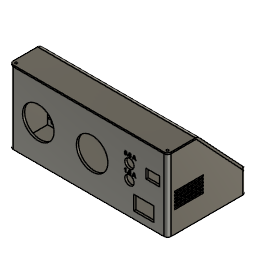
Darkroom timer box (Autodesk Fusion 360 design; units mm, degrees)
Autodesk Fusion 360 part; units mm, degrees
sketch "Sketch1" plane through (0, 0, 0) normal (0, 0, 1) x (1, 0, 0)
  line L0 (50, 125) -> (210, 125) construction
  line L1 (210, 125) -> (210, 25) construction
  line L2 (210, 25) -> (50, 25) construction
  line L3 (50, 25) -> (50, 125) construction
  line L4 (49, 225) -> (121, 225) construction
  line L5 (121, 225) -> (121, 224) construction
  line L6 (121, 224) -> (49, 224) construction
  line L7 (49, 224) -> (49, 225) construction
  line L8 (59, 224) -> (111, 224) construction
  line L9 (111, 224) -> (111, 192) construction
  line L10 (111, 192) -> (59, 192) construction
  line L11 (59, 192) -> (59, 224) construction
  line L12 (42, 225) -> (128, 225) construction
  line L13 (128, 225) -> (128, 237) construction
  line L14 (128, 237) -> (42, 237) construction
  line L15 (42, 237) -> (42, 225) construction
  line L16 (85, 240) -> (85, 190)
  line L17 (40, 130) -> (260, 130)
  line L18 (260, 130) -> (260, 20)
  line L19 (260, 20) -> (40, 20)
  line L20 (40, 20) -> (40, 130)
  line L21 (43, 127) -> (257, 127)
  line L22 (257, 127) -> (257, 23)
  line L23 (257, 23) -> (43, 23)
  line L24 (43, 23) -> (43, 127)
  line L25 (43, 115) -> (43, 120)
  line L26 (135, 120) -> (125, 120)
  line L27 (125, 120) -> (125, 127)
  line L28 (125, 127) -> (135, 127)
  line L29 (135, 127) -> (135, 120)
  line L30 (125, 30) -> (135, 30)
  line L31 (135, 30) -> (135, 23)
  line L32 (135, 23) -> (125, 23)
  line L33 (125, 23) -> (125, 30)
  line L34 (43, 35) -> (43, 30)
  line L35 (135, 126) -> (125, 126)
  line L36 (135, 24) -> (125, 24)
  circle A0 centre (44.5, 125.5) radius 1.5
  circle A1 centre (44.5, 125.5) radius 4
  circle A2 centre (255.5, 125.5) radius 1.5
  circle A3 centre (255.5, 125.5) radius 4
  line L37 (361, 251.0202) -> (361, 2.9798)
  circle A4 centre (44.5, 24.5) radius 1.5
  circle A5 centre (44.5, 24.5) radius 4
  circle A6 centre (255.5, 24.5) radius 1.5
  circle A7 centre (255.5, 24.5) radius 4
  line L38 (361, 150.0202) -> (361, -98.0202)
  line L39 (205, 70) -> (215, 70)
  line L40 (215, 70) -> (215, 80)
  line L41 (215, 80) -> (205, 80)
  line L42 (205, 80) -> (205, 70)
  line L43 (55, 70) -> (43, 70)
  line L44 (43, 70) -> (43, 80)
  line L45 (43, 80) -> (55, 80)
  line L46 (55, 80) -> (55, 70)
  line L47 (48, 70) -> (48, 80)
  line L48 (211, 70) -> (211, 80)
  point P0 (150, 75)
  dimension "d1" = 160
  dimension "d2" = 100
  dimension "d10" = 3
  dimension "d11" = 220
  dimension "d12" = 110
  constraint horizontal L0
  constraint vertical L1
  constraint horizontal L2
  constraint vertical L3
  constraint horizontal L4
  constraint vertical L5
  constraint horizontal L6
  constraint vertical L7
  constraint horizontal L8
  constraint vertical L9
  constraint horizontal L10
  constraint vertical L11
  constraint coincident L6 L8.start
  constraint horizontal L12
  constraint vertical L13
  constraint horizontal L14
  constraint vertical L15
  constraint perpendicular L10 L16
  constraint horizontal L17
  constraint vertical L18
  constraint horizontal L19
  constraint vertical L20
  constraint vertical L25
  constraint coincident L24 L25.end
  constraint horizontal L26
  constraint vertical L27
  constraint horizontal L28
  constraint vertical L29
  constraint coincident L21 L27.end
  constraint horizontal L30
  constraint vertical L31
  constraint horizontal L32
  constraint vertical L33
  constraint coincident L23 L31.end
  constraint vertical L34
  constraint coincident L24 L34.end
  constraint coincident L29 L35.start
  constraint coincident L27 L35.end
  constraint perpendicular L27 L35
  constraint coincident L31 L36.start
  constraint coincident L33 L36.end
  constraint perpendicular L33 L36
  constraint horizontal L39
  constraint vertical L40
  constraint horizontal L41
  constraint vertical L42
  constraint horizontal L43
  constraint vertical L44
  constraint horizontal L45
  constraint vertical L46
  constraint coincident L24 L44.end
  constraint coincident L45 L47.end
  constraint perpendicular L45 L47
  constraint coincident L39 L48.start
  constraint coincident L41 L48.end
  constraint perpendicular L41 L48
  measures "d1" distance of L0.start L0.end
  measures "d2" distance of L0.start L2.end
  measures "d11" distance of L17.start L17.end
  measures "d12" distance of L17.start L19.end
extrude "Extrude1" add sketch "Sketch1" along normal blind 4 contours L17 L18 L19 L20 | L21 L22 L23 L24 L25 L26 L27 L29 L30 L31 L33 L34 A1 A3 A5 A7 L43 L45 L46 | L21 L27 L28 L29 L35 | L21 L24 A0 A1 | L21 L24 A1 | L26 L27 L29 L35 | L21 L22 A3 | L21 L22 A2 A3 | L21 L24 A0 | A0 | L21 L22 A2 | A2 | L22 L23 A7 | L22 L23 A6 A7 | A6 | L22 L23 A6 | L24 L43 L44 L45 L47 | L23 L31 L32 L33 L36 | L43 L45 L46 L47 | L30 L31 L33 L36 | L23 L24 A5 | L23 L24 A4 A5 | L23 L24 A4 | A4 | L39 L41 L42 L48 | L39 L40 L41 L48 makes body 1
extrude "Extrude2" add sketch "Sketch1" along normal blind 100 contours L17 L18 L19 L20 | L21 L24 A0 A1 | L21 L24 A1 | L21 L22 A3 | L21 L22 A2 A3 | L21 L24 A0 | L21 L22 A2 | L22 L23 A7 | L22 L23 A6 A7 | L22 L23 A6 | L23 L24 A5 | L23 L24 A4 A5 | L23 L24 A4 bodies 1
extrude "Extrude3" add sketch "Sketch1" along normal blind 8 from surface at 4 contours L21 L27 L28 L29 L35 | L24 L43 L44 L45 L47 | L23 L31 L32 L33 L36 | L39 L40 L41 L48 bodies 1
extrude "Extrude5" add sketch "Sketch1" along normal blind 4 from surface at 4 contours L26 L27 L29 L35 | L43 L45 L46 L47 | L30 L31 L33 L36 | L39 L41 L42 L48 bodies 1
sketch "Sketch2" plane through (0, 20, 0) normal (0, -1, 0) x (1, 0, 0)
  line L0 (40, 0) -> (260, 0)
  line L1 (260, 0) -> (260, 100)
  line L2 (40, 100) -> (40, 0)
  circle A0 centre (80, 50) radius 22
  line L3 (45, 15) -> (45, 85)
  line L4 (45, 85) -> (115, 85)
  line L5 (115, 15) -> (45, 15)
  line L6 (115, 85) -> (115, 15)
  circle A1 centre (155, 50) radius 22
  line L7 (120, 85) -> (190, 85)
  line L8 (190, 15) -> (120, 15)
  line L9 (190, 85) -> (190, 15)
  line L10 (120, 15) -> (120, 85)
  line L11 (213, 30) -> (241, 30)
  line L12 (241, 30) -> (241, 10)
  line L13 (241, 10) -> (213, 10)
  line L14 (213, 10) -> (213, 30)
  line L15 (252, 31) -> (202, 31)
  line L16 (202, 31) -> (202, 9)
  line L17 (202, 9) -> (252, 9)
  line L18 (252, 9) -> (252, 31)
  line L19 (230, 70) -> (249, 70)
  line L20 (249, 70) -> (249, 57)
  line L21 (249, 57) -> (230, 57)
  line L22 (230, 57) -> (230, 70)
  circle A2 centre (207, 64) radius 6.5
  circle A3 centre (207, 44) radius 6.5
  line L23 (202.1965, 51) -> (201.2381, 51)
  line L24 (201.2381, 51) -> (201.2381, 54.6119)
  spline S0 degree 2 poles (201.2381, 54.6119) (200.7128, 54.1207) (200, 53.8854) knots 0 0 0 1 1 1
  line L25 (200, 53.8854) -> (200, 54.7551)
  spline S1 degree 2 poles (200, 54.7551) (200.3752, 54.8779) (200.8151, 55.2207) knots 0 0 0 1 1 1
  spline S2 degree 2 poles (200.8151, 55.2207) (201.2551, 55.5634) (201.4188, 56.0205) knots 0 0 0 1 1 1
  line L26 (201.4188, 56.0205) -> (202.1965, 56.0205)
  line L27 (202.1965, 56.0205) -> (202.1965, 51)
  line L28 (203.8336, 51) -> (203.8336, 51.9584)
  line L29 (203.8336, 51.9584) -> (204.792, 51.9584)
  line L30 (204.792, 51.9584) -> (204.792, 51)
  line L31 (204.792, 51) -> (203.8336, 51)
  line L32 (205.5832, 52.2858) -> (206.5382, 52.3847)
  spline S3 degree 2 poles (206.5382, 52.3847) (206.5791, 52.0607) (206.7804, 51.8714) knots 0 0 0 1 1 1
  spline S4 degree 2 poles (206.7804, 51.8714) (206.9816, 51.6821) (207.2442, 51.6821) knots 0 0 0 1 1 1
  spline S5 degree 2 poles (207.2442, 51.6821) (207.5443, 51.6821) (207.7524, 51.926) knots 0 0 0 1 1 1
  spline S6 degree 2 poles (207.7524, 51.926) (207.9604, 52.1699) (207.9604, 52.661) knots 0 0 0 1 1 1
  spline S7 degree 2 poles (207.9604, 52.661) (207.9604, 53.1214) (207.7541, 53.3516) knots 0 0 0 1 1 1
  spline S8 degree 2 poles (207.7541, 53.3516) (207.5478, 53.5819) (207.2169, 53.5819) knots 0 0 0 1 1 1
  spline S9 degree 2 poles (207.2169, 53.5819) (206.8042, 53.5819) (206.4768, 53.2169) knots 0 0 0 1 1 1
  line L33 (206.4768, 53.2169) -> (205.6992, 53.3295)
  line L34 (205.6992, 53.3295) -> (206.1903, 55.9318)
  line L35 (206.1903, 55.9318) -> (208.7244, 55.9318)
  line L36 (208.7244, 55.9318) -> (208.7244, 55.0348)
  line L37 (208.7244, 55.0348) -> (206.9168, 55.0348)
  line L38 (206.9168, 55.0348) -> (206.7667, 54.1855)
  spline S10 degree 2 poles (206.7667, 54.1855) (207.0873, 54.3458) (207.4216, 54.3458) knots 0 0 0 1 1 1
  spline S11 degree 2 poles (207.4216, 54.3458) (208.0593, 54.3458) (208.5027, 53.882) knots 0 0 0 1 1 1
  spline S12 degree 2 poles (208.5027, 53.882) (208.9461, 53.4181) (208.9461, 52.678) knots 0 0 0 1 1 1
  spline S13 degree 2 poles (208.9461, 52.678) (208.9461, 52.0607) (208.588, 51.5764) knots 0 0 0 1 1 1
  spline S14 degree 2 poles (208.588, 51.5764) (208.1003, 50.9147) (207.234, 50.9147) knots 0 0 0 1 1 1
  spline S15 degree 2 poles (207.234, 50.9147) (206.5416, 50.9147) (206.1051, 51.2865) knots 0 0 0 1 1 1
  spline S16 degree 2 poles (206.1051, 51.2865) (205.6685, 51.6583) (205.5832, 52.2858) knots 0 0 0 1 1 1
  line L39 (215.8561, 51) -> (214.7578, 51)
  line L40 (214.7578, 51) -> (214.3213, 52.1357)
  line L41 (214.3213, 52.1357) -> (212.3226, 52.1357)
  line L42 (212.3226, 52.1357) -> (211.91, 51)
  line L43 (211.91, 51) -> (210.839, 51)
  line L44 (210.839, 51) -> (212.7865, 56)
  line L45 (212.7865, 56) -> (213.854, 56)
  line L46 (213.854, 56) -> (215.8561, 51)
  line L47 (213.9973, 52.9782) -> (213.3083, 54.8336)
  line L48 (213.3083, 54.8336) -> (212.633, 52.9782)
  line L49 (212.633, 52.9782) -> (213.9973, 52.9782)
  spline S17 degree 2 poles (201.6235, 77.0205) (202.3499, 77.0205) (202.7592, 76.502) knots 0 0 0 1 1 1
  spline S18 degree 2 poles (202.7592, 76.502) (203.2469, 75.8881) (203.2469, 74.4659) knots 0 0 0 1 1 1
  spline S19 degree 2 poles (203.2469, 74.4659) (203.2469, 73.0471) (202.7558, 72.4263) knots 0 0 0 1 1 1
  spline S20 degree 2 poles (202.7558, 72.4263) (202.3499, 71.9147) (201.6235, 71.9147) knots 0 0 0 1 1 1
  spline S21 degree 2 poles (201.6235, 71.9147) (200.8936, 71.9147) (200.4468, 72.4758) knots 0 0 0 1 1 1
  spline S22 degree 2 poles (200.4468, 72.4758) (200, 73.0368) (200, 74.4761) knots 0 0 0 1 1 1
  spline S23 degree 2 poles (200, 74.4761) (200, 75.8881) (200.4911, 76.5089) knots 0 0 0 1 1 1
  spline S24 degree 2 poles (200.4911, 76.5089) (200.897, 77.0205) (201.6235, 77.0205) knots 0 0 0 1 1 1
  spline S25 degree 2 poles (201.6235, 76.2258) (201.4495, 76.2258) (201.3131, 76.1149) knots 0 0 0 1 1 1
  spline S26 degree 2 poles (201.3131, 76.1149) (201.1767, 76.0041) (201.1016, 75.7176) knots 0 0 0 1 1 1
  spline S27 degree 2 poles (201.1016, 75.7176) (201.0027, 75.3458) (201.0027, 74.4659) knots 0 0 0 1 1 1
  spline S28 degree 2 poles (201.0027, 74.4659) (201.0027, 73.5859) (201.0914, 73.2568) knots 0 0 0 1 1 1
  spline S29 degree 2 poles (201.0914, 73.2568) (201.1801, 72.9277) (201.3148, 72.8186) knots 0 0 0 1 1 1
  spline S30 degree 2 poles (201.3148, 72.8186) (201.4495, 72.7094) (201.6235, 72.7094) knots 0 0 0 1 1 1
  spline S31 degree 2 poles (201.6235, 72.7094) (201.7974, 72.7094) (201.9338, 72.8203) knots 0 0 0 1 1 1
  spline S32 degree 2 poles (201.9338, 72.8203) (202.0703, 72.9311) (202.1453, 73.2176) knots 0 0 0 1 1 1
  spline S33 degree 2 poles (202.1453, 73.2176) (202.2442, 73.5859) (202.2442, 74.4659) knots 0 0 0 1 1 1
  spline S34 degree 2 poles (202.2442, 74.4659) (202.2442, 75.3458) (202.1555, 75.675) knots 0 0 0 1 1 1
  spline S35 degree 2 poles (202.1555, 75.675) (202.0669, 76.0041) (201.9321, 76.1149) knots 0 0 0 1 1 1
  spline S36 degree 2 poles (201.9321, 76.1149) (201.7974, 76.2258) (201.6235, 76.2258) knots 0 0 0 1 1 1
  line L50 (204.0928, 72) -> (204.0928, 72.9584)
  line L51 (204.0928, 72.9584) -> (205.0512, 72.9584)
  line L52 (205.0512, 72.9584) -> (205.0512, 72)
  line L53 (205.0512, 72) -> (204.0928, 72)
  line L54 (209.0757, 75.7756) -> (208.148, 75.6733)
  spline S37 degree 2 poles (208.148, 75.6733) (208.1139, 75.9598) (207.9707, 76.0962) knots 0 0 0 1 1 1
  spline S38 degree 2 poles (207.9707, 76.0962) (207.8274, 76.2326) (207.5989, 76.2326) knots 0 0 0 1 1 1
  spline S39 degree 2 poles (207.5989, 76.2326) (207.2954, 76.2326) (207.0856, 75.9598) knots 0 0 0 1 1 1
  spline S40 degree 2 poles (207.0856, 75.9598) (206.8759, 75.6869) (206.8213, 74.824) knots 0 0 0 1 1 1
  spline S41 degree 2 poles (206.8213, 74.824) (207.1794, 75.2469) (207.7115, 75.2469) knots 0 0 0 1 1 1
  spline S42 degree 2 poles (207.7115, 75.2469) (208.3117, 75.2469) (208.7398, 74.7899) knots 0 0 0 1 1 1
  spline S43 degree 2 poles (208.7398, 74.7899) (209.1678, 74.3329) (209.1678, 73.6098) knots 0 0 0 1 1 1
  spline S44 degree 2 poles (209.1678, 73.6098) (209.1678, 72.8424) (208.7176, 72.3786) knots 0 0 0 1 1 1
  spline S45 degree 2 poles (208.7176, 72.3786) (208.2674, 71.9147) (207.5614, 71.9147) knots 0 0 0 1 1 1
  spline S46 degree 2 poles (207.5614, 71.9147) (206.8042, 71.9147) (206.3165, 72.5031) knots 0 0 0 1 1 1
  spline S47 degree 2 poles (206.3165, 72.5031) (205.8288, 73.0914) (205.8288, 74.4318) knots 0 0 0 1 1 1
  spline S48 degree 2 poles (205.8288, 74.4318) (205.8288, 75.8063) (206.337, 76.4134) knots 0 0 0 1 1 1
  spline S49 degree 2 poles (206.337, 76.4134) (206.8452, 77.0205) (207.6569, 77.0205) knots 0 0 0 1 1 1
  spline S50 degree 2 poles (207.6569, 77.0205) (208.2265, 77.0205) (208.5999, 76.7016) knots 0 0 0 1 1 1
  spline S51 degree 2 poles (208.5999, 76.7016) (208.9734, 76.3827) (209.0757, 75.7756) knots 0 0 0 1 1 1
  spline S52 degree 2 poles (206.9031, 73.6849) (206.9031, 73.2176) (207.118, 72.9635) knots 0 0 0 1 1 1
  spline S53 degree 2 poles (207.118, 72.9635) (207.3329, 72.7094) (207.6091, 72.7094) knots 0 0 0 1 1 1
  spline S54 degree 2 poles (207.6091, 72.7094) (207.8752, 72.7094) (208.0525, 72.9175) knots 0 0 0 1 1 1
  spline S55 degree 2 poles (208.0525, 72.9175) (208.2299, 73.1255) (208.2299, 73.5996) knots 0 0 0 1 1 1
  spline S56 degree 2 poles (208.2299, 73.5996) (208.2299, 74.0873) (208.0389, 74.3141) knots 0 0 0 1 1 1
  spline S57 degree 2 poles (208.0389, 74.3141) (207.8479, 74.5409) (207.5614, 74.5409) knots 0 0 0 1 1 1
  spline S58 degree 2 poles (207.5614, 74.5409) (207.2851, 74.5409) (207.0941, 74.3244) knots 0 0 0 1 1 1
  spline S59 degree 2 poles (207.0941, 74.3244) (206.9031, 74.1078) (206.9031, 73.6849) knots 0 0 0 1 1 1
  line L55 (216.1153, 72) -> (215.0171, 72)
  line L56 (215.0171, 72) -> (214.5805, 73.1357)
  line L57 (214.5805, 73.1357) -> (212.5819, 73.1357)
  line L58 (212.5819, 73.1357) -> (212.1692, 72)
  line L59 (212.1692, 72) -> (211.0982, 72)
  line L60 (211.0982, 72) -> (213.0457, 77)
  line L61 (213.0457, 77) -> (214.1132, 77)
  line L62 (214.1132, 77) -> (216.1153, 72)
  line L63 (214.2565, 73.9782) -> (213.5675, 75.8336)
  line L64 (213.5675, 75.8336) -> (212.8922, 73.9782)
  line L65 (212.8922, 73.9782) -> (214.2565, 73.9782)
  line L66 (260, 100) -> (40, 100)
  dimension "d45" = 44
  dimension "d48" = 35
  dimension "d49" = 35
  dimension "d50" = 5
  dimension "d51" = 44
  dimension "d52" = 35
  dimension "d53" = 35
  dimension "d54" = 28
  dimension "d55" = 20
  dimension "d56" = 50
  dimension "d57" = 22
  dimension "d58" = 19
  dimension "d59" = 13
  dimension "d60" = 13
  dimension "d63" = 0
  dimension "d64" = -20
  constraint horizontal L4
  constraint vertical L6
  constraint horizontal L5
  constraint vertical L3
  constraint horizontal L7
  constraint vertical L9
  constraint horizontal L8
  constraint vertical L10
  constraint horizontal L11
  constraint vertical L12
  constraint horizontal L13
  constraint vertical L14
  constraint horizontal L15
  constraint vertical L16
  constraint horizontal L17
  constraint vertical L18
  constraint horizontal L19
  constraint vertical L20
  constraint horizontal L21
  constraint vertical L22
  measures "d45" diameter of A0
  measures "d48" distance of A0.centre L4
  measures "d49" distance of A0.centre L6
  measures "d50" distance of L2 L3
  measures "d51" diameter of A1
  measures "d52" distance of A1.centre L7
  measures "d53" distance of A1.centre L9
  measures "d54" distance of L11.start L11.end
  measures "d55" distance of L11.start L13.end
  measures "d56" distance of L15.start L15.end
  measures "d57" distance of L15.end L16.end
  measures "d58" distance of L19.start L19.end
  measures "d59" distance of L19.start L21.end
  measures "d60" diameter of A2
extrude "Extrude4" add sketch "Sketch1" along normal blind 2 from surface at 4 contours L26 L27 L29 L35 | L30 L31 L33 L36 bodies 1
extrude "Extrude6" cut sketch "Sketch2" against normal blind 3 contours A0 | A1 | L11 L12 L13 L14 | L19 L20 L21 L22 | A2 | A3 bodies 1
extrude "Extrude8" cut sketch "Sketch2" against normal blind 1 contours L23 L24 S0 L25 S1 S2 L26 L27 | L28 L29 L30 L31 | L32 S3 S4 S5 S6 S7 S8 S9 L33 L34 L35 L36 L37 L38 S10 S11 S12 S13 S14 S15 S16 | L39 L40 L41 L42 L43 L44 L45 L46 | S17 S18 S19 S20 S21 S22 S23 S24 | L50 L51 L52 L53 | L54 S37 S38 S39 S40 S41 S42 S43 S44 S45 S46 S47 S48 S49 S50 S51 | L55 L56 L57 L58 L59 L60 L61 L62 bodies 1
sketch "Sketch3" plane through (260, 0, 0) normal (1, 0, 0) x (0, 1, 0)
  line L0 (20, 0) -> (130, 0)
  line L1 (130, 0) -> (130, 100)
  line L2 (20, 100) -> (20, 0)
  line L3 (60, 100) -> (130, 25)
  line L4 (130, 25) -> (130, 100)
  line L5 (130, 25) -> (130, 28)
  line L6 (20, 100) -> (60, 100)
  line L7 (20, 102.0527) -> (62.1878, 102.0527)
  line L8 (62.1878, 102.0527) -> (130, 29.3968)
  line L9 (20, 102.0527) -> (20, 100)
  line L10 (130, 25) -> (130, 29.3968)
  line L11 (130, 100) -> (20, 100)
  constraint coincident L1 L3.end
  constraint coincident L1.end L4.end
  constraint coincident L4 L5.end
  constraint coincident L2.start L6.start
  constraint coincident L1 L8.end
extrude "Extrude7" cut sketch "Sketch3" against normal blind 220 contours L1 L3 L4 L5 L8 L10 L11 | L1 L4 L8 L11 bodies 1
extrude "Extrude9" add sketch "Sketch3" against normal blind 220 separate body contours L6 L7 L8 L9 L11 | L1 L3 L4 L5 L8 L10 L11 makes body 2
sketch "Sketch4" plane through (0, 0, 102.0527) normal (0, 0, 1) x (-1, 0, 0)
  line L0 (-260, -20) -> (-260, -62.1878)
  line L1 (-260, -62.1878) -> (-40, -62.1878)
  line L2 (-40, -62.1878) -> (-40, -20)
  line L3 (-40, -20) -> (-260, -20)
  circle A0 centre (-255.5, -24.5) radius 1.5
  circle A1 centre (-44.5, -24.5) radius 1.5
  circle A2 centre (-255.5, -125.5) radius 1.5
  circle A3 centre (-44.5, -125.5) radius 1.5
  dimension "d90" = 211
  dimension "d91" = -101
extrude "Extrude10" cut sketch "Sketch4" against normal blind 75 contours A0 | A1 | A2 | A3 bodies 2
sketch "Sketch5" plane through (0, 84.1409, 78.5315) normal (0, 0.731055, 0.682318) x (-1, 0, 0)
  line L0 (-260, 32.1742) -> (-260, -67.2107)
  line L1 (-260, -67.2107) -> (-40, -67.2107)
  line L2 (-40, -67.2107) -> (-40, 32.1742)
  line L3 (-40, 32.1742) -> (-260, 32.1742)
  circle A0 centre (-202.5, -9.986) radius 6
  circle A1 centre (-167.5, -9.986) radius 6
  circle A2 centre (-132.5, -9.986) radius 6
  circle A3 centre (-97.5, -9.986) radius 6
  circle A4 centre (-167.5, -39.986) radius 6
  circle A5 centre (-132.5, -39.986) radius 6
  line L4 (-180.5, 24.014) -> (-119.5, 24.014)
  line L5 (-119.5, 24.014) -> (-119.5, 10.014)
  line L6 (-119.5, 10.014) -> (-180.5, 10.014)
  line L7 (-180.5, 10.014) -> (-180.5, 24.014)
  circle A6 centre (-114.5, 12.014) radius 2.5
  circle A7 centre (-114.5, 21.014) radius 2.5
  circle A8 centre (-190.5, 20.986) radius 2.5
  circle A9 centre (-190.5, 11.986) radius 2.5
  circle A10 centre (-114.5, 21.014) radius 5
  circle A11 centre (-114.5, 12.014) radius 5
  circle A12 centre (-190.5, 20.986) radius 5
  circle A13 centre (-190.5, 11.986) radius 5
  line L8 (-118.5, 9.014) -> (-181.5, 9.014)
  line L9 (-181.5, 9.014) -> (-181.5, 25.014)
  line L10 (-181.5, 25.014) -> (-118.5, 25.014)
  line L11 (-118.5, 25.014) -> (-118.5, 9.014)
  line L12 (-187, 27) -> (-187, 5)
  ellipse E0 centre (-44.5, -60.6155) end of major axis (-44.5, -62.8139) minor radius 1.5
  ellipse E1 centre (-255.5, -60.6155) end of major axis (-255.5, -62.8139) minor radius 1.5
  dimension "d94" = 12
  dimension "d97" = 35
  dimension "d98" = -30
  dimension "d99" = 61
  dimension "d100" = 14
  dimension "d101" = 22
  dimension "d102" = 22
  dimension "d103" = 20
  dimension "d104" = 5
  dimension "d106" = 5
  dimension "d107" = 9
  dimension "d108" = 2
  dimension "d109" = 5
  dimension "d110" = 5
  dimension "d111" = 76
  dimension "d112" = 5
  dimension "d113" = 9
  dimension "d114" = 57.5
  dimension "d115" = 57.5
  dimension "d116" = 5
  dimension "d117" = 10
  dimension "d118" = 10
  dimension "d119" = 10
  dimension "d120" = 10
  dimension "d121" = 10
  dimension "d122" = 10
  dimension "d123" = -1
  constraint horizontal L4
  constraint vertical L5
  constraint horizontal L6
  constraint vertical L7
  constraint concentric A7 A10
  constraint concentric A6 A11
  constraint concentric A8 A12
  constraint concentric A9 A13
  constraint vertical L12
  measures "d94" diameter of A0
  measures "d99" distance of L4.start L4.end
  measures "d100" distance of L4.start L6.end
  measures "d101" distance of A0.centre L7
  measures "d102" distance of A3.centre L5
  measures "d103" distance of A1.centre L6
  measures "d104" diameter of A6
  measures "d106" diameter of A7
  measures "d107" distance of A6.centre A7.centre
  measures "d108" distance of L6 A6.centre
  measures "d109" distance of L5 A6.centre
  measures "d110" diameter of A8
  measures "d111" distance of A7.centre A8.centre
  measures "d112" diameter of A9
  measures "d113" distance of A8.centre A9.centre
  measures "d114" distance of L0 A0.centre
  measures "d115" distance of L2 A3.centre
  measures "d116" distance of L5 A7.centre
  measures "d117" distance of L7 A9.centre
  measures "d118" distance of L7 A8.centre
  measures "d119" diameter of A10
  measures "d120" diameter of A11
  measures "d121" diameter of A12
  measures "d122" diameter of A13
extrude "Extrude11" add sketch "Sketch5" against normal blind 4 from surface at -3 contours A10 A11 L11 | A10 A11 L11 | A10 A11 | A12 A13 L12 | A12 A13 | A12 A13 L12 picked at (-118, 21.014) picked at (-118, 12.014) picked at (-187.3333, 20.986) picked at (-187.3333, 11.986) bodies 2
extrude "Extrude12" cut sketch "Sketch5" against normal blind 5 contours A0 | A1 | A2 | A3 | A4 | A5 | L4 L5 L6 L7 A10 A11 L8 L9 L10 L11 | L4 L5 L6 L7 | L5 A10 A11 L11 | A10 L11 | A11 L11 bodies 2
fillet "Fillet1" radius 5 8 edges at (40, 20, 50) (40, 130, 12.5) (260, 130, 12.5) (260, 20, 50) (40, 20, 101.0263) (40, 130, 27.1984) (260, 130, 27.1984) (260, 20, 101.0263) on bodies 1 2
fillet "Fillet2" radius 7.5 1 edges at (150, 62.1878, 102.0527) on bodies 2
sketch "Sketch7" plane through (260, 0, 0) normal (1, 0, 0) x (0, 1, 0)
  line L0 (25, 100) -> (25, 0)
  line L1 (25, 0) -> (125, 0)
  line L2 (125, 0) -> (125, 30.3571)
  line L3 (125, 30.3571) -> (60, 100)
  line L4 (60, 100) -> (25, 100)
  line L5 (30, 50) -> (70, 50)
  line L6 (70, 50) -> (70, 52)
  line L7 (70, 52) -> (30, 52)
  line L8 (30, 52) -> (30, 50)
  line L9 (30, 46) -> (70, 46)
  line L10 (30, 48) -> (30, 46)
  line L11 (70, 46) -> (70, 48)
  line L12 (70, 48) -> (30, 48)
  line L13 (30, 42) -> (70, 42)
  line L14 (30, 44) -> (30, 42)
  line L15 (70, 42) -> (70, 44)
  line L16 (70, 44) -> (30, 44)
  line L17 (30, 38) -> (70, 38)
  line L18 (30, 40) -> (30, 38)
  line L19 (70, 38) -> (70, 40)
  line L20 (70, 40) -> (30, 40)
  line L21 (30, 34) -> (70, 34)
  line L22 (30, 36) -> (30, 34)
  line L23 (70, 34) -> (70, 36)
  line L24 (70, 36) -> (30, 36)
  line L25 (30, 30) -> (70, 30)
  line L26 (30, 32) -> (30, 30)
  line L27 (70, 30) -> (70, 32)
  line L28 (70, 32) -> (30, 32)
  dimension "d141" = 40
  dimension "d142" = 2
  dimension "d145" = 0
  dimension "d146" = -20
  constraint horizontal L5
  constraint vertical L6
  constraint horizontal L7
  constraint vertical L8
  measures "d141" distance of L5.start L5.end
  measures "d142" distance of L5.start L7.end
extrude "Extrude14" cut sketch "Sketch7" along normal mid plane 14 contours L5 L6 L7 L8 | L9 L10 L11 L12 | L13 L14 L15 L16 | L17 L18 L19 L20 | L21 L22 L23 L24 | L25 L26 L27 L28 bodies 1
equation "wallThickness = 3 mm"
equation "d10 = wallThickness"
equation "buttonDiameter = 12 mm"
equation "d25 = wallHeight"
equation "wallHeight = 100 mm"
equation "d94 = buttonDiameter"
equation "d101 = d102"
equation "d114 = d115"
equation "d116 = d109"
equation "d117 = d118"
named bodies: "box", "lid"
